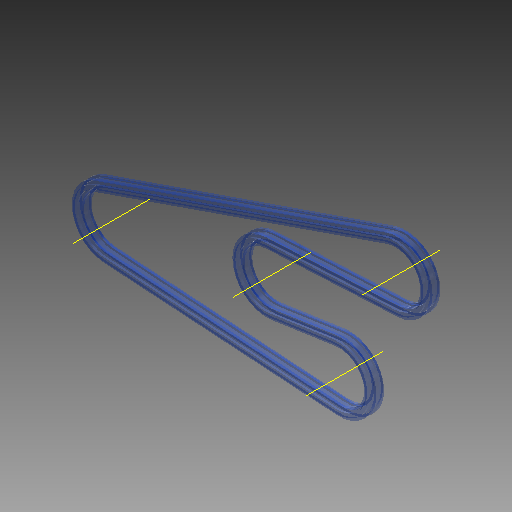
# Autodesk Inventor part: Roller Chain
Saved by Autodesk Inventor 2017 (Build 210142000, 142)
## iProperties
Created: 2016-10-08
Part Number: Roller Chain
Material: Generic
Document SubType Name: Modeling
Designer: gus
Density: 1 g/cm^3
Appearance: Clear - Blue
Mass: 23.536 g
Surface Area: 237.721 cm^2
Volume: 23.536 cm^3
CustomPartVersion: 1
Author: gus
Autodesk Inventor part; units mm, degrees
ref_plane "Work Plane2" through (-98.8573, -20.95, 0) normal (-1, 0, 0) x (0, 0, 1)
ref_plane "Work Plane3" through (44.5845, -30.4224, 0) normal (0.9920776, 0.1256263, 0) x (0, 0, 1)
ref_plane "Work Plane4" through (0, 0, 0) normal (0.995421, -0.0955883, 0) x (0, 0, 1)
ref_plane "Work Plane5" through (79.1543, 40.5989, 0) normal (0.9621844, 0.272399, 0) x (0, 0, 1)
sketch "Path" plane through (0, 0, 0) normal (0, 0, 1) x (1, 0, 0)
  arc A0 (-104.8321, -3.6697) -> (-100.0621, -39.1944) centre (-98.8573, -20.95) ccw
  arc A1 (43.3797, -48.6668) -> (41.9321, -12.3317) centre (44.5845, -30.4224) ccw
  arc A2 (-0.9192, 18.261) -> (2.6524, -18.0907) centre (0, 0) ccw
  arc A3 (80.0735, 22.3379) -> (73.1795, 57.8792) centre (79.1543, 40.5989) ccw
  line L0 (73.1795, 57.8792) -> (-104.8321, -3.6697)
  line L1 (-100.0621, -39.1944) -> (43.3797, -48.6668)
  line L2 (41.9321, -12.3317) -> (2.6524, -18.0907)
  line L3 (-0.9192, 18.261) -> (80.0735, 22.3379)
  constraints: 8 end point, 8 point on circle, 4 centre point
ref_plane "Section Plane" through (-104.8321, -3.6697, 0) normal (-0.9451017, -0.3267764, 0) x (0, 0, 1)
sketch "Section Sketch" plane through (-104.8321, -3.6697, 0) normal (-0.9451017, -0.3267764, 0) x (0, 0, 1)
  line L0 (-4.318, -1.1494) -> (4.318, -1.1494)
  line L1 (4.318, -1.1494) -> (4.318, 1.1494)
  line L2 (4.318, 1.1494) -> (-4.318, 1.1494)
  line L3 (-4.318, 1.1494) -> (-4.318, -1.1494)
  line L4 (-1.5875, -1.651) -> (1.5875, -1.651)
  line L5 (1.5875, -1.651) -> (1.5875, 1.651)
  line L6 (1.5875, 1.651) -> (-1.5875, 1.651)
  line L7 (-1.5875, 1.651) -> (-1.5875, -1.651)
  line L8 (-1.5875, 0) -> (1.5875, 0) construction
  line L9 (-3.1115, -2.9972) -> (-1.5875, -2.9972)
  line L10 (-1.5875, -2.9972) -> (-1.5875, 2.9972)
  line L11 (-1.5875, 2.9972) -> (-3.1115, 2.9972)
  line L12 (-3.1115, 2.9972) -> (-3.1115, -2.9972)
  line L13 (1.5875, -2.9972) -> (3.1115, -2.9972)
  line L14 (3.1115, -2.9972) -> (3.1115, 2.9972)
  line L15 (3.1115, 2.9972) -> (1.5875, 2.9972)
  line L16 (1.5875, 2.9972) -> (1.5875, -2.9972)
  line L17 (-4.318, 0) -> (4.318, 0) construction
  point P0 (0, 0)
  point P1 (0, 0)
  dimension "d21" = 2.2987
  dimension "d22" = 3.302
  dimension "d23" = 3.175
  dimension "d24" = 1.524
  dimension "d31" = 5.9944
  dimension "d32" = 8.636
  constraints: 36 end point, 8 midpoint, 8 parallel, 4 horizontal, 4 perpendicular, 3 collinear, 1 coincident, 1 other
  measures "d21" distance between parallel lines of L2 L0
  measures "d22" distance between parallel lines of L6 L4
  measures "d23" distance between parallel lines of L5 L7
  measures "d24" distance between parallel lines of L12 L10
  measures "d31" distance between parallel lines of L11 L9
  measures "d32" distance between parallel lines of L1 L3
sweep "Solid" add profiles "Section Sketch" path "Path"
pattern_of_one "Strand Pattern"
equation "\"d21\" = da_d2"
equation "\"d22\" = da_d1"
equation "\"d23\" = da_b1"
equation "\"d24\" = da_t1 + da_t2"
equation "\"d30\" = da_pt"
equation "\"da_p\" = 6.35"
equation "\"da_b1\" = 3.175"
equation "\"da_h2\" = 5.9944"
equation "\"da_h3\" = 5.207"
equation "\"da_d1\" = 3.302"
equation "\"da_d2\" = 2.2987"
equation "\"da_pt\" = 6.4008"
equation "\"da_b\" = 8.636"
equation "\"da_t1\" = 0.762"
equation "\"da_t2\" = 0.762"
body "Solid1"
